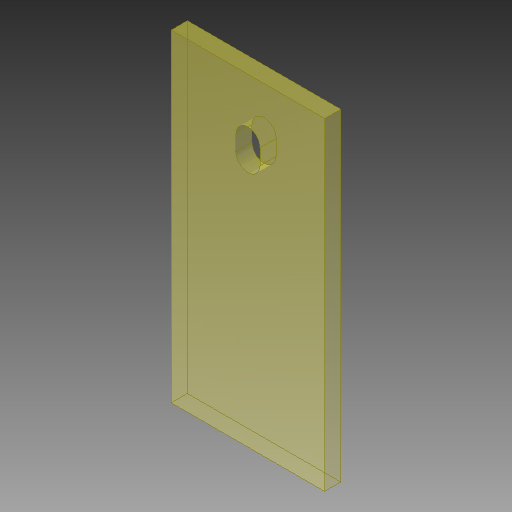
# Autodesk Inventor part: support plate
Saved by Autodesk Inventor 2018.1 (Build 221171000, 171)
## iProperties
Created: 2017-07-29
Part Number: support plate
Material: PVC-Piping
Document SubType Name: Modeling
Designer: Tom
Density: 1.4 g/cm^3
Appearance: Clear - Yellow
Mass: 2128 g
Surface Area: 1756 cm^2
Volume: 1520 cm^3
Author: Tom
Autodesk Inventor part; units mm, degrees
ref_plane "YZ Plane" through (0, 0, 0) normal (1, 0, 0) x (0, 1, 0)
ref_plane "XZ Plane" through (0, 0, 0) normal (0, 1, 0) x (-1, 0, 0)
ref_plane "XY Plane" through (0, 0, 0) normal (0, 0, 1) x (1, 0, 0)
sketch "Sketch1" plane through (0, 0, 0) normal (0, 0, 1) x (1, 0, 0)
  line L0 (0, 0) -> (190, 0)
  line L1 (190, 0) -> (190, 400)
  line L2 (190, 400) -> (0, 400)
  line L3 (0, 400) -> (0, 0)
  dimension "d0" = 190
  dimension "d1" = 400
  constraints: 8 end point, 2 parallel, 1 horizontal, 1 perpendicular
  measures "d0" distance of L2.end L1.end
  measures "d1" distance of L1.end L0.end
extrude "Extrusion1" add sketch "Sketch1" along normal blind 20
sketch "Sketch2" plane through (0, 0, 20) normal (0, 0, 1) x (1, 0, 0)
  circle A0 centre (95, 328.575) radius 5 construction
  circle A1 centre (95, 309.525) radius 5 construction
  arc A2 (110, 328.575) -> (80, 328.575) centre (95, 328.575) ccw construction
  arc A3 (80, 309.525) -> (110, 309.525) centre (95, 309.525) ccw construction
  line L0 (95, 309.525) -> (110, 309.525) construction
  line L1 (95, 309.525) -> (80, 309.525) construction
  line L2 (80, 309.525) -> (80, 328.575)
  line L3 (110, 328.575) -> (110, 309.525)
  arc A4 (110, 328.575) -> (80, 328.575) centre (95, 328.575) ccw
  arc A5 (80, 309.525) -> (110, 309.525) centre (95, 309.525) ccw
  point P0 (0, 0)
  dimension "d4" = 15
  dimension "d5" = 15
  dimension "d6" = 180
  constraints: 8 end point, 8 point on circle, 4 centre point, 4 coincident, 1 parallel, 1 vertical
  measures "d4" radius of A2
  measures "d5" radius of A3
  measures "d6" angle of L1 L0
extrude "Extrusion2" cut sketch "Sketch2" against normal blind 20
equation "\"d0\" = maxw - 4 * nutdist"
equation "\"d1\" = maxh"
equation "\"d2\" = supt"
equation "\"d7\" = supt"
equation "\"maxh\" = 400"
equation "\"lcsd\" = 19.05"
equation "\"lcwd1\" = 25"
equation "\"lcwd2\" = 34"
equation "\"lch1\" = 39"
equation "\"lcwd3\" = 43"
equation "\"dia1\" = 6"
equation "\"td\" = 18"
equation "\"bhh\" = 6"
equation "\"sw\" = 25"
equation "\"sh\" = 31"
equation "\"spacert\" = 2"
equation "\"supt\" = 20"
equation "\"pvct\" = 5"
equation "\"dia3\" = 8"
equation "\"dia4\" = 11"
equation "\"tankl\" = 379"
equation "\"play\" = 9"
equation "\"holeh\" = 26"
equation "\"surroundt\" = 5"
equation "\"slack\" = 0.5"
equation "\"play2\" = 3"
equation "\"diacucl\" = 32"
equation "\"diaoverflow\" = 25"
equation "\"diawater\" = 25"
equation "\"diaph\" = 32"
equation "\"diaair\" = 32"
equation "\"diasurroundhole\" = 42"
equation "\"diagrate\" = 12"
equation "\"gratespacing\" = 12.02082"
equation "\"sidedist\" = 13.9375"
equation "\"bottomdist\" = 9.6355"
equation "\"diahcl\" = 32"
equation "\"bracketwtop\" = 6"
equation "\"bracketwbottom\" = 6"
equation "\"nett\" = 1"
equation "\"nethole\" = 16"
equation "\"nettop\" = 7"
equation "\"netside\" = 3.5"
equation "\"netholespacing\" = 2"
equation "\"diaetape\" = 32"
equation "\"maxw\" = 350"
equation "\"nutdist\" = 40"
body "Solid1"
